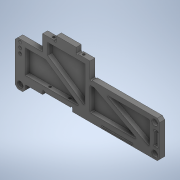
# Autodesk Inventor part: Cockpit_vertical_frame_03
Saved by Autodesk Inventor 2020 (Build 240168000, 168)
## iProperties
Created: 2021-04-12
Part Number: Cockpit_vertical_frame_03
Material: アセタール樹脂、黒
Document SubType Name: Modeling
Designer: Masato Kubotera
Density: 1.425 g/cm^3
Appearance: 滑らか - 黒
Mass: 26.6371 g
Surface Area: 177.414 cm^2
Volume: 18.6927 cm^3
Description: POM T5
d0: 145.000 mm
d1: 53.000 mm
d2: 75.000 mm
d3: 16.000 mm
d4: 2.500 mm
d5: 3.100 mm
d6: 2.500 mm
d7: 5.000 mm
d12: 20.000 mm
d14: 5.000 mm
d15: 1.050 mm
d16: 1.050 mm
d53: 1.050 mm
d54: 1.050 mm
d55: 1.050 mm
d56: 1.050 mm
d59: 5.000 mm
d60: 0.00 deg
d107: 30.000 mm
d108: 1.500 mm
d109: 0.050 mm
d110: 0.050 mm
d114: 0.050 mm
d115: 0.050 mm
d116: 30.000 mm
d118: 5.000 mm
d120: 132.500 mm
d124: 15.000 mm
d125: 0.050 mm
d126: 0.050 mm
d127: 1.050 mm
d128: 1.050 mm
d129: 1.050 mm
d130: 1.050 mm
d132: 30.000 mm
d134: 3.000 mm
d135: 2.500 mm
d140: 5.000 mm
d144: 5.000 mm
d146: 5.000 mm
d147: 20.000 mm
d152: 1.050 mm
d169: 6.000 mm
d170: 2.000 mm
d171: 0.00 deg
d172: 2.500 mm
d176: 20.000 mm
d185: 5.000 mm
d186: 5.000 mm
d187: 5.000 mm
d190: 8.000 mm
d191: 5.000 mm
d192: 5.000 mm
d193: 5.000 mm
d196: 2.500 mm
d197: 1.000 mm
d198: 0.500 mm
d199: 0.00 deg
d17: 70.000 mm
d74: 37.000 mm
d148: 130.000 mm
Author: Masato Kubotera
Title: Cockpit_vertical_frame_03
Autodesk Inventor part; units mm, degrees
ref_plane "YZ Plane" through (0, 0, 0) normal (1, 0, 0) x (0, 1, 0)
ref_plane "XZ Plane" through (0, 0, 0) normal (0, 1, 0) x (-1, 0, 0)
ref_plane "XY Plane" through (0, 0, 0) normal (0, 0, 1) x (1, 0, 0)
sketch "スケッチ2" plane through (-42.95, -23.5, 0) normal (0, -1, 0) x (1, 0, 0)
  line L0 (0, 0) -> (25.9, 5) construction
  line L1 (0, 5) -> (25.9, 5) projected
  line L2 (12.95, 5) -> (12.95, 0) construction
  line L3 (0, 0) -> (25.9, 0) projected
  line L4 (0, 0) -> (0, 5) projected
  line L5 (0, 2.5) -> (25.9, 2.5) construction
  line L6 (25.9, 0) -> (25.9, 5) projected
  point P0 (42.95, 0)
  point P1 (2.95, 2.5)
  point P2 (22.95, 2.5)
  dimension "d176" = 20
  constraints: 6 end point, 4 midpoint, 1 coincident, 1 point on line, 1 symmetric about line
  measures "d176" distance of point (22.95, 2.5) point (2.95, 2.5)
sketch "スケッチ1" plane through (0, 0, 0) normal (0, 0, 1) x (1, 0, 0)
  line L0 (-72.5, 26.5) -> (-45, 26.5) construction
  line L1 (72.5, 26.5) -> (72.5, 10.5) construction
  line L2 (-72.5, -26.5) -> (-72.5, 10.5)
  line L3 (-72.5, 26.5) -> (72.5, -26.5) construction
  line L4 (72.5, 26.5) -> (-72.5, -26.5) construction
  line L5 (2.5, 26.5) -> (2.5, 10.5)
  line L6 (2.5, 10.5) -> (4.6, 10.5) construction
  line L7 (2.5, 26.5) -> (72.5, 26.5) construction
  line L8 (72.5, 10.5) -> (72.5, -26.5)
  line L9 (70, 10.5) -> (70, -26) construction
  circle A0 centre (67.5, 5.5) radius 1.55
  line L10 (-31.25, 26.5) -> (-31.25, 31.5)
  line L11 (-31.25, 31.5) -> (-11.25, 31.5)
  line L12 (-11.25, 31.5) -> (-11.25, 26.5)
  line L13 (-31.25, 26.5) -> (-11.25, 26.5) construction
  line L14 (-11.25, 26.5) -> (-9.15, 26.5) construction
  arc A1 (-33.35, 26.5) -> (-31.25, 26.5) centre (-32.3, 26.5) ccw
  arc A2 (-11.25, 26.5) -> (-9.15, 26.5) centre (-10.2, 26.5) ccw
  line L15 (-33.35, 26.5) -> (-31.25, 26.5) construction
  line L16 (-9.15, 26.5) -> (2.5, 26.5)
  line L17 (-45.05, -23.5) -> (-42.95, -23.5) construction
  arc A3 (-42.95, -23.5) -> (-45.05, -23.5) centre (-44, -23.5) ccw
  arc A4 (-14.95, -23.5) -> (-17.05, -23.5) centre (-16, -23.5) ccw
  line L18 (-42.95, -23.5) -> (-17.05, -23.5)
  line L19 (-17.05, -23.5) -> (-14.95, -23.5) construction
  line L20 (15, -23.5) -> (45, -23.5) construction
  line L21 (45, -23.5) -> (45, -25) construction
  line L22 (45, -25) -> (15, -25) construction
  line L23 (15, -25) -> (15, -23.5) construction
  line L24 (15, -23.5) -> (45, -25) construction
  line L25 (45, -23.5) -> (15, -25) construction
  line L26 (14.95, -23.45) -> (45.05, -23.45)
  line L27 (45.05, -23.45) -> (45.05, -25.05) construction
  line L28 (45.05, -25.05) -> (14.95, -25.05)
  line L29 (14.95, -25.05) -> (14.95, -23.45) construction
  line L30 (14.95, -23.45) -> (45.05, -25.05) construction
  line L31 (45.05, -23.45) -> (14.95, -25.05) construction
  line L32 (-45, -23.5) -> (-45, -26.5) construction
  line L33 (-15, -23.5) -> (-15, -26.5) construction
  line L34 (72.5, -8) -> (-72.5, -8) construction
  line L35 (70, -0.5) -> (67.5, -0.5) construction
  line L36 (67.5, -0.5) -> (67.5, -15.5) construction
  line L37 (67.5, -15.5) -> (70, -15.5) construction
  line L38 (70, -15.5) -> (70, -0.5) construction
  line L39 (70, -0.5) -> (67.5, -15.5) construction
  line L40 (67.5, -0.5) -> (70, -15.5) construction
  line L41 (67.45, -0.45) -> (70.05, -0.45)
  line L42 (70.05, -0.45) -> (70.05, -2.55) construction
  line L43 (70.05, -15.55) -> (67.45, -15.55)
  line L44 (67.45, -15.55) -> (67.45, -13.45) construction
  line L45 (67.45, -0.45) -> (70.05, -15.55) construction
  line L46 (70.05, -0.45) -> (67.45, -15.55) construction
  arc A5 (67.45, -0.45) -> (67.45, -2.55) centre (67.45, -1.5) ccw
  arc A6 (70.05, -2.55) -> (70.05, -0.45) centre (70.05, -1.5) ccw
  arc A7 (67.45, -13.45) -> (67.45, -15.55) centre (67.45, -14.5) ccw
  arc A8 (70.05, -15.55) -> (70.05, -13.45) centre (70.05, -14.5) ccw
  line L47 (67.45, -2.55) -> (67.45, -0.45) construction
  line L48 (67.45, -13.45) -> (67.45, -2.55)
  line L49 (70.05, -13.45) -> (70.05, -15.55) construction
  line L50 (70.05, -2.55) -> (70.05, -13.45)
  arc A9 (14.95, -23.45) -> (14.95, -25.05) centre (14.95, -24.25) ccw
  arc A10 (45.05, -25.05) -> (45.05, -23.45) centre (45.05, -24.25) ccw
  circle A11 centre (67.5, -21.5) radius 1.55
  line L51 (-72.5, -26.5) -> (-62.5, -26.5) construction
  line L52 (-15, -26.5) -> (72.5, -26.5)
  line L53 (-45, -26.5) -> (-15, -26.5) construction
  line L54 (-70, 26) -> (-70, -26.5) construction
  line L55 (-65, 26.5) -> (-65, -26.5) construction
  arc A12 (2.5, 10.5) -> (4.6, 10.5) centre (3.55, 10.5) ccw
  line L56 (4.6, 10.5) -> (72.5, 10.5)
  circle A13 centre (67.5, 5.5) radius 3
  circle A14 centre (67.5, -21.5) radius 3
  line L57 (2.5, 5.5) -> (2.5, -18.5)
  line L58 (2.5, -18.5) -> (51.8308, -18.5)
  line L59 (51.8308, -18.5) -> (6.5905, 5.5)
  line L60 (17.2597, 5.5) -> (62.5, 5.5)
  line L61 (62.5, 5.5) -> (62.5, -18.5)
  line L62 (62.5, -18.5) -> (17.2597, 5.5)
  line L63 (-62.5, -18.5) -> (-6.9355, -18.5)
  line L64 (-6.9355, -18.5) -> (-42.1079, 5.5)
  line L65 (-2.5, 21.5) -> (-2.5, -15.4734)
  line L66 (-2.5, -15.4734) -> (-40, 10.1148)
  line L67 (2.5, 10.5) -> (2.5, -26.5) construction
  line L68 (6.5905, 5.5) -> (2.5, 5.5)
  line L69 (2.5, 10.5) -> (72.2455, -26.5) construction
  circle A15 centre (-67.5, -29) radius 1.25
  circle A16 centre (-67.5, -29) radius 3
  circle A17 centre (-67.5, -2) radius 1.5
  circle A18 centre (-67.5, 3) radius 1.5
  circle A19 centre (-67.5, 8) radius 1.5
  line L70 (-67.5, 26.5) -> (-67.5, -26.5) construction
  line L71 (-45.05, -23.5) -> (-45.05, -26.5)
  line L72 (-14.95, -23.5) -> (-14.95, -26.5)
  line L73 (-45, 26.5) -> (-45, 21.5)
  line L74 (-45, 10.5) -> (-72.5, 10.5)
  line L75 (-62.5, 5.5) -> (-42.1079, 5.5)
  line L76 (-40, 21.5) -> (-40, 10.1148)
  line L77 (-72.5, -26.5) -> (-72.5, -34)
  line L78 (-72.5, -34) -> (-62.5, -34)
  line L79 (-62.5, -26.5) -> (-62.5, -34)
  line L80 (-62.5, -26.5) -> (-45, -26.5)
  line L81 (-45, 26.5) -> (-33.35, 26.5)
  line L82 (-45, 21.5) -> (-45, 10.5)
  line L83 (-62.5, 5.5) -> (-62.5, -18.5)
  line L84 (-2.5, -18.5) -> (-45, 10.5) construction
  line L85 (-45.05, 21.5) -> (-45, 21.5)
  line L86 (-40, 21.5) -> (-2.5, 21.5)
  line L87 (-72.5, 10.5) -> (-72.5, 26.5) construction
  point P0 (0, 0)
  point P1 (30, -24.25)
  point P2 (68.75, -8)
  point P3 (-60, 14.6054)
  point P4 (-46.25, 11.0112)
  point P5 (-54.1904, 10.5)
  point P6 (-45.5266, 10.5)
  dimension "d0" = 145
  dimension "d1" = 53
  dimension "d2" = 75
  dimension "d3" = 16
  dimension "d4" = 2.5
  dimension "d5" = 3.1
  dimension "d6" = 2.5
  dimension "d7" = 5
  dimension "d12" = 20
  dimension "d14" = 5
  dimension "d15" = 1.05
  dimension "d16" = 1.05
  dimension "d17" = 70
  dimension "d55" = 1.05
  dimension "d56" = 1.05
  dimension "d74" = 37
  dimension "d107" = 30
  dimension "d108" = 1.5
  dimension "d109" = 0.05
  dimension "d110" = 0.05
  dimension "d116" = 30
  dimension "d124" = 15
  dimension "d125" = 0.05
  dimension "d126" = 0.05
  dimension "d127" = 1.05
  dimension "d128" = 1.05
  dimension "d129" = 1.05
  dimension "d130" = 1.05
  dimension "d132" = 30
  dimension "d134" = 3
  dimension "d135" = 2.5
  dimension "d146" = 5
  dimension "d147" = 20
  dimension "d152" = 1.05
  dimension "d169" = 6
  dimension "d186" = 5
  dimension "d187" = 5
  dimension "d190" = 8
  dimension "d192" = 5
  dimension "d193" = 5
  dimension "d196" = 2.5
  dimension "d200" = 2.5
  dimension "d201" = 6
  dimension "d205" = 2.5
  dimension "d206" = 3
  dimension "d207" = 3
  dimension "d208" = 3
  dimension "d209" = 2.5
  dimension "d211" = 5
  dimension "d212" = 5
  dimension "d213" = 0.05
  dimension "d214" = 0.05
  dimension "d215" = 2.5
  dimension "d216" = 5
  dimension "d217" = 2.5
  dimension "d220" = 18.5
  dimension "d222" = 16
  dimension "d225" = 13.75
  dimension "d226" = 27.5
  dimension "d227" = 5
  dimension "d228" = 5
  dimension "d233" = 7.5
  dimension "d234" = 2.5
  dimension "d235" = 2.5
  constraints: 176 end point, 51 perpendicular, 29 point on line, 25 parallel, 24 midpoint, 22 point on circle, 21 horizontal, 20 centre point, 8 vertical, 4 collinear, 4 symmetric about line, 2 coincident, 2 other
  measures "d0" distance of L3.end L2.start
  measures "d1" distance of L1.start L3.end
  measures "d2" distance between parallel lines of L2 L5
  measures "d3" distance of L5.start L5.end
  measures "d4" distance between parallel lines of L8 L9
  measures "d5" diameter of A0
  measures "d6" distance from line of L9 A0.centre
  measures "d7" distance from line of L6 A0.centre
  measures "d12" distance of L10.end L11.end
  measures "d14" distance between parallel lines of L11 L0
  measures "d15" radius of A1
  measures "d16" radius of A2
  measures "d17" distance of L5.end L1.end
  measures "d55" radius of A3
  measures "d56" radius of A4
  measures "d74" distance of L1.end L3.end
  measures "d107" distance of L21.end L22.end
  measures "d108" distance of L20.end L21.end
  measures "d109" distance between parallel lines of L29 L23
  measures "d110" distance between parallel lines of L26 L20
  measures "d116" distance between parallel lines of L32 L33
  measures "d124" distance of L37.end L35.start
  measures "d125" distance between parallel lines of L41 L35
  measures "d126" distance between parallel lines of L42 L38
  measures "d127" radius of A5
  measures "d128" radius of A6
  measures "d129" radius of A8
  measures "d130" radius of A7
  measures "d132" distance between parallel lines of L23 L33
  measures "d134" distance between parallel lines of L51 L18
  measures "d135" distance between parallel lines of L2 L54
  measures "d146" distance between parallel lines of L54 L55
  measures "d147" distance between parallel lines of L55 L32
  measures "d152" radius of A12
  measures "d169" diameter of A13
  measures "d186" distance between parallel lines of L5 L65
  measures "d187" distance between parallel lines of L66 L64
  measures "d190" distance between parallel lines of L51 L63
  measures "d192" distance between parallel lines of L59 L62
  measures "d193" distance between parallel lines of L56 L60
  measures "d196" distance between parallel lines of L59 L69
  measures "d200" diameter of A15
  measures "d201" diameter of A16
  measures "d205" horizontal distance of A15.centre L54.start
  measures "d206" diameter of A17
  measures "d207" diameter of A18
  measures "d208" diameter of A19
  measures "d209" distance of L70.end L54.end
  measures "d211" distance of A17.centre A18.centre
  measures "d212" distance of A18.centre A19.centre
  measures "d213" distance between parallel lines of L71 L32
  measures "d214" distance between parallel lines of L72 L33
  measures "d215" distance between parallel lines of L8 L38
  measures "d216" distance between parallel lines of L36 L61
  measures "d217" distance between parallel lines of L36 L38
  measures "d220" distance from line of A19.centre L0
  measures "d222" distance between parallel lines of L74 L0
  measures "d225" distance between parallel lines of L12 L5
  measures "d226" distance between parallel lines of L2 L73
  measures "d227" distance between parallel lines of L73 L76
  measures "d228" distance between parallel lines of L75 L74
  measures "d233" distance between parallel lines of L78 L51
  measures "d234" distance between parallel lines of L64 L84
  measures "d235" distance between parallel lines of L55 L83
extrude "押し出し1" add sketch "スケッチ1" along normal blind 5 contours L2 L74 L82 L73 L81 A1 L10 L11 L12 A2 L16 L5 A12 L56 L8 L52 L72 A4 L18 A3 L71 L80 L79 L78 L77
extrude "押し出し2" add sketch "スケッチ1" along normal blind 2 contours A13 | A14 | A16
hole "穴1" at (-40, -23.5, 2.5) at (-20, -23.5, 2.5) direction (0, 1, 0) diameter 2.459 depth 5 thread size "M3x0.5" class "6H" standard "ISO Metric profile"
chamfer "面取り1" distance 2.5 angle 45 5 edges at (72.5, -26.5, 2.5) (72.5, 10.5, 2.5) (-72.5, -34, 2.5) (-72.5, 10.5, 2.5) (-62.5, -34, 2.5)
fillet "フィレット2" radius 1 11 edges at (-6.9355, -18.5, 2.5) (-2.5, -15.4734, 2.5) (2.5, -18.5, 2.5) (2.5, 5.5, 2.5) (6.5905, 5.5, 2.5) (17.2597, 5.5, 2.5) (62.5, 5.5, 2.5) (62.5, -18.5, 2.5) (51.8308, -18.5, 2.5) (-45, 10.5, 2.5) (-62.5, -26.5, 2.5)
extrude "押し出し4" add sketch "スケッチ1" along normal blind 0.5 contours L68 L59 L58 L57 | L60 L61 L62 | L83 L75 L64 L63 | L65 L66 L76 L86
sketch "スケッチ9" plane through (-45, 26.5, 0) normal (0, 1, 0) x (1, 0, 0)
  line L0 (33.75, 0) -> (33.75, -5) projected
  line L1 (13.75, 0) -> (13.75, -5) projected
  line L2 (33.75, 0) -> (13.75, 0) projected
  line L3 (47.5, 0) -> (35.85, 0) projected
  point P0 (45, 0)
  point P1 (8.75, -2.5)
  point P2 (38.75, -2.5)
  dimension "d237" = 20
  dimension "d238" = 30
  dimension "d239" = 5
  dimension "d240" = 2.5
  dimension "d241" = 2.5
  measures "d237" distance between parallel lines of L0 L1
  measures "d238" distance of point (38.75, -2.5) point (8.75, -2.5)
  measures "d239" distance from line of point (8.75, -2.5) L1
  measures "d240" distance from line of point (8.75, -2.5) L2
  measures "d241" distance from line of point (38.75, -2.5) L3
hole "穴6" at (-36.25, 26.5, 2.5) at (-6.25, 26.5, 2.5) direction (0, -1, 0) diameter 2.459 depth 5 thread size "M3x0.5" class "6H" standard "ISO Metric profile"
equation "\"d16\" = d15"
equation "\"d55\" = d54"
equation "\"d56\" = d55"
equation "\"d53\" = d15"
equation "\"d54\" = d53"
